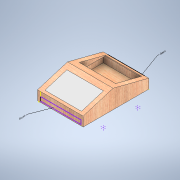
# Autodesk Inventor part: Part1proj
Saved by Autodesk Inventor 2020 (Build 240168000, 168)
## iProperties
Created: 2020-03-23
Part Number: Part1proj
Material: Wood (Birch)
Document SubType Name: Modeling
Designer: Manish
Density: 0.55 g/cm^3
Appearance: Birch - Natural Polished
Author: Manish
Autodesk Inventor part; units mm, degrees
ref_plane "YZ Plane" through (0, 0, 0) normal (1, 0, 0) x (0, 1, 0)
ref_plane "XZ Plane" through (0, 0, 0) normal (0, 1, 0) x (-1, 0, 0)
ref_plane "XY Plane" through (0, 0, 0) normal (0, 0, 1) x (1, 0, 0)
sketch "Sketch1" plane through (0, 0, 0) normal (0, 1, 0) x (-1, 0, 0)
  line L0 (7.9003, 23.0254) -> (-242.0997, 23.0254)
  line L1 (-242.0997, 23.0254) -> (-242.0997, -336.9746)
  line L2 (-242.0997, -336.9746) -> (7.9003, -336.9746)
  line L3 (7.9003, -336.9746) -> (7.9003, 23.0254)
  point P0 (0, 0)
  dimension "d0" = 250
  dimension "d1" = 360
  constraints: 8 end point, 2 parallel, 1 horizontal, 1 perpendicular
  measures "d0" distance of L2.end L1.end
  measures "d1" distance of L1.end L0.end
extrude "Extrusion1" add sketch "Sketch1" along normal blind 52
shell "Shell1" thickness 15 removed faces 1 at (158.7664, 52, -96.9746)
sketch3d "3D Sketch5"
sketch "Sketch8" plane through (242.0997, 0, 23.0254) normal (1, 0, 0) x (0, 0, -1)
  line L0 (0, 52) -> (164.1703, 102.1919)
  line L1 (0, 52) -> (171.6715, 52) construction
  line L2 (0, 52) -> (360, 52) projected
  line L3 (164.1703, 102.1919) -> (360, 52)
  line L4 (360, 52) -> (0, 52)
  point P0 (23.0254, 0)
  dimension "d27" = 17
  constraints: 8 end point, 1 collinear, 1 equal length, 1 horizontal
  measures "d27" angle of L1 L0
extrude "Extrusion4" add sketch "Sketch8" against normal up to surface (250 mm away)
sketch "Sketch9" plane through (-7.9003, 102.1919, -141.1449) normal (0, 0.9686887, -0.2482786) x (1, 0, 0)
  line L0 (15, 187.6292) -> (235, 187.6292) projected
  line L1 (225, 40.9807) -> (25, 40.9807)
  line L2 (25, 40.9807) -> (25, 187.6292)
  line L3 (25, 187.6292) -> (225, 187.6292)
  line L4 (225, 187.6292) -> (225, 40.9807)
  line L5 (250, 202.1596) -> (250, 0) projected
  line L6 (0, 202.1596) -> (0, 0) projected
  point P0 (7.9003, -111.3534)
  point P1 (225, 187.6292)
  dimension "d30" = 25
  dimension "d31" = 25
  constraints: 8 end point, 2 parallel, 1 horizontal, 1 perpendicular, 1 point on line
  measures "d30" distance between parallel lines of L4 L5
  measures "d31" distance between parallel lines of L6 L2
extrude "Extrusion5" cut sketch "Sketch9" against normal blind 30
sketch "Sketch10" plane through (242.0997, 0, -336.9746) normal (0, 0, -1) x (-1, 0, 0)
  line L0 (225, 52) -> (25, 52) projected
  line L1 (0, 0) -> (250, 0) projected
  line L2 (25, 52) -> (226.6576, 52)
  line L3 (226.6576, 52) -> (226.6576, 0)
  line L4 (226.6576, 0) -> (25, 0)
  line L5 (25, 0) -> (25, 52)
  point P0 (242.0997, 0)
  constraints: 8 end point, 2 parallel, 1 horizontal, 1 perpendicular, 1 point on line
sketch "Sketch11" plane through (-7.9003, 0, 23.0254) normal (0, 0, 1) x (1, 0, 0)
  line L0 (15, 15) -> (15, 52) projected
  line L1 (15, 28.3801) -> (237.0279, 28.3801)
  line L2 (237.0279, 28.3801) -> (237.0279, 6.6777)
  line L3 (237.0279, 6.6777) -> (15, 6.6777)
  line L4 (15, 6.6777) -> (15, 28.3801)
  point P0 (7.9003, 0)
  constraints: 8 end point, 2 parallel, 1 horizontal, 1 perpendicular, 1 point on line
sketch "Sketch12" plane through (-7.9003, 52, 23.0254) normal (0, 0.9563048, 0.2923717) x (1, 0, 0)
  line L0 (235, 14.3446) -> (15, 14.3446) projected
  line L1 (26.6812, 140.3694) -> (227.0114, 140.3694)
  line L2 (227.0114, 140.3694) -> (227.0114, 14.3446)
  line L3 (227.0114, 14.3446) -> (26.6812, 14.3446)
  line L4 (26.6812, 14.3446) -> (26.6812, 140.3694)
  point P0 (7.9003, 6.8159)
  constraints: 8 end point, 2 parallel, 1 horizontal, 1 perpendicular, 1 point on line
extrude "Extrusion6" add sketch "Sketch12" against normal blind 2 separate body
body "Solid1"
body "Solid4"
